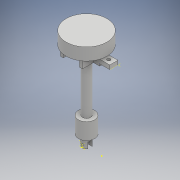
# Autodesk Inventor part: CosaCuello
Saved by Autodesk Inventor 2017 SP1 (Build 210196100, 196)
## iProperties
Part Number: CosaCuello
Material: Genérico
Document SubType Name: Modeling
Designer: Juan
Density: 1 g/cm^3
Appearance: Valor por defecto
Author: Juan
Autodesk Inventor part; units mm, degrees
sketch "Boceto1" plane through (0, 0, 0) normal (1, 0, 0) x (0, 1, 0)
  line L0 (5.2272, 23.4487) -> (5.2272, 13.4487)
  line L1 (15.2272, 13.4487) -> (15.2272, 23.4487)
  line L2 (5.2272, 13.4487) -> (15.2272, 13.4487)
  line L3 (5.2272, 23.4487) -> (15.2272, 23.4487)
  line L4 (15.2272, 23.4487) -> (20.2272, 23.4487)
  line L5 (20.2272, 23.4487) -> (20.2272, 53.4487)
  line L6 (20.2272, 53.4487) -> (15.2272, 53.4487)
  line L7 (15.2272, 53.4487) -> (15.2272, 213.4487)
  line L8 (15.2272, 213.4487) -> (5.2272, 213.4487)
  line L9 (5.2272, 213.4487) -> (5.2272, 53.4487)
  line L10 (5.2272, 23.4487) -> (0.2272, 23.4487)
  line L11 (0.2272, 23.4487) -> (0.2272, 53.4487)
  line L12 (0.2272, 53.4487) -> (5.2272, 53.4487)
  point P0 (0, 0)
  dimension "d0" = 10
  dimension "d1" = 10
  dimension "d2" = 10
  dimension "d74" = 5
  dimension "d75" = 30
  dimension "d76" = 160
  dimension "d77" = 5
  constraints: 26 end point, 7 perpendicular, 3 horizontal, 1 point on line, 1 vertical
  measures "d0" distance of L1.end L0.start
  measures "d1" distance of L0.start L0.end
  measures "d2" distance of L1.start L1.end
  measures "d74" distance of L1.end L4.end
  measures "d75" distance of L4.end L5.end
  measures "d76" distance of L6.end L7.end
  measures "d77" distance of L0.start L10.end
revolve "Revolución1" add sketch "Boceto1" angle 360 about axis through (0, 5.2272, 23.4487) along (0, 0, -1) contours L3 L1 L2 L0
ref_plane "Plano de trabajo1" through (0, 5.2272, 13.4487) normal (0, 0, -1) x (-1, 0, 0)
sketch "Boceto10" plane through (0, 5.2272, 13.4487) normal (0, 0, -1) x (-1, 0, 0)
  line L0 (0, 0) -> (0, -5) construction
  line L1 (0, 0) -> (0, 5) construction
  circle A0 centre (0, 0) radius 10 projected
  line L2 (8.525, -5.2272) -> (-8.525, -5.2272)
  line L3 (8.525, 5.2272) -> (-8.525, 5.2272)
  arc A1 (-8.525, -5.2272) -> (8.525, -5.2272) centre (0, 0) ccw
  arc A2 (8.525, 5.2272) -> (-8.525, 5.2272) centre (0, 0) ccw
  point P0 (0, -5.2272)
  dimension "d50" = 5
  dimension "d51" = 5
  constraints: 8 end point, 8 point on circle, 2 centre point, 2 vertical, 1 concentric, 1 horizontal, 1 parallel
  measures "d50" distance of L0.start L0.end
  measures "d51" distance of L0.start L1.end
extrude "Extrusión2" add sketch "Boceto10" along normal blind 15 contours L3 A0 | A0 L2
ref_plane "Plano de trabajo6" through (-8.525, -5.5, 13.4487) normal (0, 1, 0) x (1, 0, 0)
sketch "Boceto12" plane through (-8.525, -5.5, 13.4487) normal (0, 1, 0) x (1, 0, 0)
  line L0 (17.0501, 15) -> (0, 15) construction
  line L1 (17.0501, 15) -> (0, 0) construction
  line L2 (0, 15) -> (17.0501, 0) construction
  point P0 (8.525, 13.4487)
  constraints: 4 end point
hole "Agujero4" at (0.0012, 0, 5.9481) direction (0, -1, 0) diameter 5 end through all
hole "Agujero5" at (0.0198, 10.4545, 5.9266) direction (0, 1, 0) diameter 5 end through all
ref_plane "Plano de trabajo7" through (0, 5.2272, 23.4487) normal (0, 0, 1) x (1, 0, 0)
sketch "Boceto13" plane through (0, 5.2272, 23.4487) normal (0, 0, 1) x (1, 0, 0)
  circle A0 centre (0, 0) radius 20
  point P0 (0, -5.2272)
  dimension "d79" = 40
  constraints: 1 centre point
  measures "d79" diameter of A0
extrude "Extrusión3" add sketch "Boceto13" along normal blind 40
ref_plane "Plano de trabajo8" through (0, 5.2272, 63.4487) normal (0, 0, 1) x (1, 0, 0)
sketch "Boceto14" plane through (0, 5.2272, 63.4487) normal (0, 0, 1) x (1, 0, 0)
  circle A0 centre (0, 0) radius 10
  point P0 (0, -5.2272)
  dimension "d83" = 20
  constraints: 1 centre point
  measures "d83" diameter of A0
extrude "Extrusión4" add sketch "Boceto14" along normal blind 150
ref_plane "Plano de trabajo9" through (0, 5.2272, 213.4487) normal (0, 0, 1) x (1, 0, 0)
sketch "Boceto15" plane through (0, 5.2272, 213.4487) normal (0, 0, 1) x (1, 0, 0)
  circle A0 centre (0, 0) radius 50
  point P0 (0, -5.2272)
  dimension "d87" = 100
  constraints: 1 centre point
  measures "d87" diameter of A0
extrude "Extrusión5" add sketch "Boceto15" along normal blind 30
ref_plane "Plano de trabajo10" through (0, 5.2272, 213.4487) normal (0, 0, -1) x (-1, 0, 0)
sketch "Boceto20" plane through (0, 5.2272, 213.4487) normal (0, 0, -1) x (-1, 0, 0)
  circle A0 centre (0, 0) radius 10 construction
  line L0 (0, 0) -> (-20, 0) construction
  line L1 (-20, 0) -> (-20, 10) construction
  line L2 (-20, 0) -> (-20, -10) construction
  line L3 (0, 0) -> (20, 0) construction
  line L4 (20, 0) -> (20, -10) construction
  line L5 (20, 0) -> (20, 10) construction
  line L6 (20, -10) -> (20, -37)
  line L7 (20, -37) -> (27, -37)
  line L8 (27, -37) -> (27, -10)
  line L9 (27, -10) -> (20, -10)
  line L10 (-20, -10) -> (-20, -37)
  line L11 (-20, -37) -> (-27, -37)
  line L12 (-27, -37) -> (-27, -10)
  line L13 (-27, -10) -> (-20, -10)
  line L14 (-20, 10) -> (-20, 37)
  line L15 (-20, 37) -> (-27, 37)
  line L16 (-27, 37) -> (-27, 10)
  line L17 (-27, 10) -> (-20, 10)
  line L18 (20, 10) -> (20, 37)
  line L19 (20, 37) -> (27, 37)
  line L20 (27, 37) -> (27, 10)
  line L21 (20, 10) -> (27, 10)
  point P0 (0, -5.2272)
  dimension "d123" = 20
  dimension "d124" = 10
  dimension "d125" = 10
  dimension "d126" = 20
  dimension "d127" = 10
  dimension "d128" = 10
  dimension "d129" = 27
  dimension "d130" = 7
  dimension "d131" = 27
  dimension "d132" = 7
  dimension "d133" = 27
  dimension "d134" = 27
  constraints: 44 end point, 9 perpendicular, 9 point on line, 4 vertical, 2 horizontal
  measures "d123" distance of L0.start L0.end
  measures "d124" distance of L0.end L1.end
  measures "d125" distance of L0.end L2.end
  measures "d126" distance of L0.start L3.end
  measures "d127" distance of L3.end L4.end
  measures "d128" distance of L3.end L5.end
  measures "d129" distance of L4.end L6.end
  measures "d130" distance of L6.end L7.end
  measures "d131" distance of L2.end L10.end
  measures "d132" distance of L10.end L11.end
  measures "d133" distance of L1.end L14.end
  measures "d134" distance of L5.end L18.end
extrude "Extrusión9" add sketch "Boceto20" along normal blind 20
ref_plane "Plano de trabajo13" through (-27, 15.2272, 213.4487) normal (-1, 0, 0) x (0, 0, 1)
sketch "Boceto21" plane through (-27, 15.2272, 213.4487) normal (-1, 0, 0) x (0, 0, 1)
  line L0 (-20, 0) -> (-20, 27) construction
  line L1 (-20, 27) -> (-20, 7) construction
  line L2 (-20, 7) -> (-7, 7) construction
  line L3 (0, 40) -> (0, -60) construction
  line L4 (0, 0) -> (0, 27) construction
  line L5 (0, 7) -> (-13, 7) construction
  line L6 (-13, 7) -> (-7, 7)
  line L7 (-13, 7) -> (-13, 3)
  line L8 (-13, 3) -> (-7, 3)
  line L9 (-7, 3) -> (-7, 7)
  point P0 (-213.4487, -15.2272)
  dimension "d138" = 20
  dimension "d139" = 13
  dimension "d140" = 13
  dimension "d141" = 4
  constraints: 14 end point, 4 perpendicular, 3 point on line, 1 collinear
  measures "d138" distance of L0.end L1.end
  measures "d139" distance of L1.end L2.end
  measures "d140" distance of L5.start L5.end
  measures "d141" distance of L5.end L7.end
extrude "Extrusión10" cut sketch "Boceto21" against normal blind 20
ref_plane "Plano de trabajo14" through (-27, -31.7728, 213.4487) normal (-1, 0, 0) x (0, 0, 1)
sketch "Boceto22" plane through (-27, -31.7728, 213.4487) normal (-1, 0, 0) x (0, 0, 1)
  line L0 (-20, 0) -> (-20, 27) construction
  line L1 (-20, 0) -> (-20, 20) construction
  line L2 (-20, 20) -> (-7, 20) construction
  line L3 (0, 27) -> (0, 0) construction
  line L4 (0, 20) -> (-13, 20) construction
  line L5 (-13, 20) -> (-7, 20)
  line L6 (-7, 20) -> (-7, 24)
  line L7 (-7, 24) -> (-13, 24)
  line L8 (-13, 24) -> (-13, 20)
  point P0 (-213.4487, 31.7728)
  dimension "d145" = 20
  dimension "d146" = 13
  dimension "d147" = 13
  constraints: 14 end point, 3 point on line, 2 perpendicular, 1 collinear, 1 horizontal, 1 vertical
  measures "d145" distance of L0.start L1.end
  measures "d146" distance of L1.end L2.end
  measures "d147" distance of L4.start L4.end
extrude "Extrusión11" cut sketch "Boceto22" against normal blind 20
sketch "Boceto23" plane through (0, 5.2272, 213.4487) normal (0, 0, -1) x (-1, 0, 0)
  circle A0 centre (0, 0) radius 10 projected
  line L0 (0, 0) -> (-27, 0) construction
  line L1 (-27, 10) -> (-27, 37) projected
  line L2 (-27, -10) -> (-20, -10) projected
  line L3 (-27, 10) -> (-27, -10)
  line L4 (-27, -10) -> (-42, -10)
  line L5 (-42, -10) -> (-42, 10)
  line L6 (-42, 10) -> (-27, 10)
  point P0 (0, -5.2272)
  dimension "d152" = 27
  dimension "d153" = 15
  constraints: 10 end point, 3 perpendicular, 1 horizontal, 1 vertical
  measures "d152" distance of L0.start L0.end
  measures "d153" distance of L2.start L4.end
extrude "Extrusión12" add sketch "Boceto23" along normal blind 20 contours L3 L4 L5 L6
sketch "Boceto24" plane through (42, -4.7728, 213.4487) normal (1, 0, 0) x (0, 0, -1)
  point P0 (213.4487, 4.7728)
ref_plane "Plano de trabajo15" through (42, -4.7728, 213.4487) normal (1, 0, 0) x (0, 0, -1)
sketch "Boceto25" plane through (42, -4.7728, 213.4487) normal (1, 0, 0) x (0, 0, -1)
  line L0 (20, 0) -> (20, 20) projected
  line L1 (0, 0) -> (20, 0) projected
  line L2 (20, 0) -> (15, 0) construction
  line L3 (0, 0) -> (5, 0) construction
  line L4 (0, -40) -> (0, 60) construction
  line L5 (0, 20) -> (5, 20) construction
  line L6 (20, 20) -> (15, 20) construction
  line L7 (0, 20) -> (20, 20) construction
  line L8 (15, 20) -> (15, 0)
  line L9 (15, 20) -> (5, 20)
  line L10 (5, 0) -> (5, 20)
  line L11 (15, 0) -> (5, 0)
  point P0 (213.4487, 4.7728)
  dimension "d158" = 5
  dimension "d159" = 5
  constraints: 16 end point, 4 point on line, 2 collinear, 1 horizontal, 1 perpendicular, 1 vertical
  measures "d158" distance of L0.start L2.end
  measures "d159" distance of L1.start L3.end
extrude "Extrusión13" add sketch "Boceto25" along normal blind 25
sketch "Boceto26" plane through (42, -4.7728, 198.4487) normal (0, 0, -1) x (-1, 0, 0)
  point P0 (42, 4.7728)
ref_plane "Plano de trabajo16" through (42, -4.7728, 198.4487) normal (0, 0, -1) x (-1, 0, 0)
sketch "Boceto27" plane through (42, -4.7728, 198.4487) normal (0, 0, -1) x (-1, 0, 0)
  line L0 (0, 20) -> (0, 0) construction
  line L1 (0, 0) -> (-25, 20) construction
  line L2 (0, 20) -> (-25, 20) construction
  line L3 (-25, 0) -> (-25, 20) construction
  line L4 (0, 20) -> (-25, 0) construction
  point P0 (42, 4.7728)
  constraints: 4 end point
hole "Agujero6" at (54.4978, 5.2307, 198.4487) direction (0, 0, 1) diameter 8 end through all
